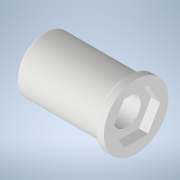
# Autodesk Inventor part: Hülse2
Saved by Autodesk Inventor 2022 (Build 260153000, 153)
## iProperties
Created: 2022-01-02
Part Number: Hülse2
Material: Generisch
Document SubType Name: Modeling
Designer: Jan
Density: 1 g/cm^3
Appearance: Vorgabe
Author: Jan
Autodesk Inventor part; units mm, degrees
ref_plane "YZ Plane" through (0, 0, 0) normal (1, 0, 0) x (0, 1, 0)
ref_plane "XZ Plane" through (0, 0, 0) normal (0, 1, 0) x (-1, 0, 0)
ref_plane "XY Plane" through (0, 0, 0) normal (0, 0, 1) x (1, 0, 0)
sketch "Skizze1" plane through (0, 0, 0) normal (0, 0, 1) x (1, 0, 0)
  line L0 (20, -3) -> (22, -3)
  line L1 (13, -3) -> (20, -3)
  line L2 (13, 3) -> (20, 3)
  line L3 (13, -3) -> (13, 3) projected
  line L4 (20, 3) -> (22, 3)
  line L5 (22, 3.5) -> (23, 3.5)
  line L6 (22, -3.5) -> (22, 3.5) projected
  line L7 (22, -3.5) -> (23, -3.5)
  line L8 (23, 3.5) -> (23, -3.5) projected
  line L9 (13, 0) -> (25, 0)
  line L10 (13, 0) -> (13, 3)
  line L11 (22, 3) -> (22, 3.5)
  line L12 (23, 3.5) -> (23, 0)
  point P0 (0, 0)
  dimension "d24" = 10
  dimension "d25" = 1
  dimension "d26" = 7
  dimension "d27" = 6
  constraints: 20 end point, 7 horizontal, 2 collinear, 2 midpoint, 1 parallel, 1 point on line, 9 other
  measures "d24" distance between parallel lines of L3 L8
  measures "d25" distance between parallel lines of L6 L8
  measures "d26" diameter of L5 L9
  measures "d27" distance between parallel lines of L1 L2
revolve "Umdrehung1" add sketch "Skizze1" angle 360 about axis through (13, 0, 0) along (1, 0, 0) contours L9 L3 L2 L4 L6 | L6 L5 L8 L9
chamfer "Fase1" distance 0.2 angle 45 1 edges at (13, -3, 0)
chamfer "Fase2" distance 0.2 angle 45 1 edges at (22, -3.5, 0)
sketch "Skizze3" plane through (23, 0, 0) normal (1, 0, 0) x (0, 0, -1)
  line L0 (1.25, 2.1651) -> (2.5, 0)
  line L1 (2.5, 0) -> (1.25, -2.1651)
  line L2 (1.25, -2.1651) -> (-1.25, -2.1651)
  line L3 (-1.25, -2.1651) -> (-2.5, 0)
  line L4 (-2.5, 0) -> (-1.25, 2.1651)
  line L5 (-1.25, 2.1651) -> (1.25, 2.1651)
  point P0 (0, 0)
  point P1 (0, 0)
  dimension "d28" = 2.5
  constraints: 12 end point, 1 coincident, 13 other
  measures "d28" distance of L4.end L0.start
sketch "Skizze4" plane through (22, 0, 0) normal (-1, 0, 0) x (0, 0, 1)
  point P0 (0, 0)
hole "Bohrung2" at (22, 0, 0) direction (-1, 0, 0) diameter 3 end through all
extrude "Extrusion1" cut sketch "Skizze3" against normal up to surface (1 mm away)
chamfer "Fase3" distance 0.2 angle 45 1 edges at (22, 0, 1.5)
chamfer "Fase4" distance 0.2 angle 45 6 edges at (23, 2.1651, 0) (23, 1.0825, -1.875) (23, -1.0825, -1.875) (23, -2.1651, 0) (23, -1.0825, 1.875) (23, 1.0825, 1.875)
